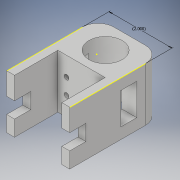
# Autodesk Inventor part: Vertical Seeder Rod spacer
Saved by Autodesk Inventor 2017 (Build 210142000, 142)
## iProperties
Created: 2017-05-29
Part Number: Vertical Seeder Rod spacer
Material: Generic
Document SubType Name: Modeling
Designer: Jon
Density: 1 g/cm^3
Appearance: Default
Author: Jon
Autodesk Inventor part; units mm, degrees
ref_plane "YZ Plane" through (0, 0, 0) normal (1, 0, 0) x (0, 1, 0)
ref_plane "XZ Plane" through (0, 0, 0) normal (0, 1, 0) x (-1, 0, 0)
ref_plane "XY Plane" through (0, 0, 0) normal (0, 0, 1) x (1, 0, 0)
sketch "Sketch1" plane through (0, 0, 0) normal (0, 0, 1) x (1, 0, 0)
  line L0 (-15.24, 10.0753) -> (16.51, 10.0753)
  line L1 (16.51, 10.0753) -> (16.51, -15.3247)
  line L2 (16.51, -15.3247) -> (-15.24, -15.3247)
  line L3 (-15.24, -15.3247) -> (-15.24, 10.0753)
  circle A0 centre (-11.43, 6.2653) radius 1.905
  circle A1 centre (-11.43, -6.4347) radius 1.905
  circle A2 centre (12.7, 6.2653) radius 1.905
  circle A3 centre (12.7, -6.4347) radius 1.905
  point P0 (0, 0)
  dimension "d0" = 31.75
  dimension "d1" = 25.4
  dimension "d10" = 3.81
  dimension "d11" = 8.89
  dimension "d12" = 3.81
  dimension "d13" = 3.81
  dimension "d14" = 8.89
  dimension "d15" = 3.81
  dimension "d16" = 3.81
  dimension "d17" = 3.81
  dimension "d18" = 3.81
  dimension "d19" = 3.81
  dimension "d20" = 3.81
  dimension "d21" = 3.81
  dimension "d22" = 8.89
  constraints: 8 end point, 4 centre point, 2 parallel, 1 horizontal, 1 perpendicular
  measures "d0" distance of L0.start L0.end
  measures "d1" distance of L0.end L1.end
  measures "d10" diameter of A0
  measures "d12" distance from line of L0 A0.centre
  measures "d13" distance from line of L3 A0.centre
  measures "d14" distance from line of L2 A1.centre
  measures "d15" diameter of A2
  measures "d16" diameter of A1
  measures "d17" diameter of A3
  measures "d18" distance from line of L3 A1.centre
  measures "d19" distance from line of L0 A2.centre
  measures "d20" distance from line of L1 A2.centre
  measures "d21" distance from line of L1 A3.centre
  measures "d22" distance from line of L2 A3.centre
extrude "Extrusion1" add sketch "Sketch1" along normal blind 6.35
sketch "Sketch2" plane through (0, 0, 6.35) normal (0, 0, 1) x (1, 0, 0)
  line L0 (-24.765, 16.4253) -> (26.035, 16.4253)
  line L1 (26.035, 16.4253) -> (26.035, -21.6747)
  line L2 (26.035, -21.6747) -> (-24.765, -21.6747)
  line L3 (-24.765, -21.6747) -> (-24.765, 16.4253)
  line L4 (16.51, -15.3247) -> (16.51, 10.0753) projected
  line L5 (-15.24, 10.0753) -> (-15.24, -15.3247) projected
  line L6 (16.51, 10.0753) -> (-15.24, 10.0753) projected
  point P0 (0, 0)
  dimension "d25" = 50.8
  dimension "d26" = 38.1
  dimension "d27" = 9.525
  dimension "d29" = 9.525
  dimension "d30" = 6.35
  constraints: 8 end point, 2 parallel, 1 horizontal, 1 perpendicular
  measures "d25" distance of L0.start L0.end
  measures "d26" distance of L0.end L1.end
  measures "d27" distance between parallel lines of L4 L1
  measures "d29" distance between parallel lines of L3 L5
  measures "d30" distance between parallel lines of L6 L0
extrude "Extrusion2" add sketch "Sketch2" along normal blind 6.35
sketch "Sketch3" plane through (0, 0, 6.35) normal (0, 0, -1) x (-1, 0, 0)
  line L0 (24.765, -21.6747) -> (24.765, 16.4253) projected
  circle A0 centre (11.43, 6.2653) radius 1.905 projected
  line L1 (24.765, 16.4253) -> (-26.035, 16.4253) projected
  circle A1 centre (11.43, -6.4347) radius 1.905 projected
  line L2 (-26.035, -21.6747) -> (24.765, -21.6747) projected
  line L3 (-26.035, 16.4253) -> (-26.035, -21.6747) projected
  point P0 (0, 0)
  point P1 (-12.7, -6.4347)
  point P2 (-12.7, 6.2653)
  dimension "d33" = 13.335
  dimension "d34" = 10.16
  dimension "d35" = 13.335
  dimension "d36" = 15.24
  dimension "d37" = 13.335
  dimension "d38" = 10.16
  dimension "d39" = 15.24
  dimension "d40" = 13.335
  constraints: 2 coincident
  measures "d33" distance from line of L0 A0.centre
  measures "d34" distance from line of L1 A0.centre
  measures "d35" distance from line of L0 A1.centre
  measures "d36" distance from line of L2 A1.centre
  measures "d37" distance from line of L3 point (-12.7, 6.265)
  measures "d38" distance from line of L1 point (-12.7, 6.265)
  measures "d39" distance from line of L2 point (-12.7, -6.435)
  measures "d40" distance from line of L3 point (-12.7, -6.435)
hole "Hole1" at (-11.43, 6.2653, 6.35) at (-11.43, -6.4347, 6.35) at (12.7, -6.4347, 6.35) at (12.7, 6.2653, 6.35) direction (0, 0, 1) diameter 3.81 end through all
sketch "Sketch4" plane through (0, 0, 12.7) normal (0, 0, 1) x (1, 0, 0)
  line L0 (26.035, 16.4253) -> (26.035, -21.6747) projected
  line L1 (26.035, 16.4253) -> (19.685, 16.4253)
  line L2 (19.685, 16.4253) -> (19.685, -21.6747)
  line L3 (19.685, -21.6747) -> (26.035, -21.6747)
  line L4 (26.035, -21.6747) -> (26.035, 16.4253)
  line L5 (-24.765, 16.4253) -> (26.035, 16.4253) projected
  line L6 (-24.765, 16.4253) -> (-18.415, 16.4253)
  line L7 (-18.415, 16.4253) -> (-18.415, -21.6747)
  line L8 (-18.415, -21.6747) -> (-24.765, -21.6747)
  line L9 (-24.765, -21.6747) -> (-24.765, 16.4253)
  point P0 (0, 0)
  dimension "d48" = 6.35
  dimension "d49" = 6.35
  constraints: 16 end point, 4 parallel, 2 horizontal, 2 perpendicular, 1 point on line
  measures "d48" distance of L2.end L3.end
  measures "d49" distance of L7.end L8.end
extrude "Extrusion3" add sketch "Sketch4" along normal blind 34.925
sketch "Sketch5" plane through (26.035, -21.6747, 6.35) normal (1, 0, 0) x (0, 0, -1)
  line L0 (-41.2903, 25.4) -> (-28.2305, 25.4)
  line L1 (-28.2305, 25.4) -> (-28.2305, 12.7)
  line L2 (-28.2305, 12.7) -> (-41.2903, 12.7)
  line L3 (-41.2903, 12.7) -> (-41.2903, 25.4)
  line L4 (0, 38.1) -> (-41.275, 38.1) projected
  point P0 (6.35, 21.6747)
  dimension "d52" = 12.7
  dimension "d53" = 12.7
  constraints: 8 end point, 2 parallel, 1 horizontal, 1 perpendicular
  measures "d52" distance between parallel lines of L4 L0
  measures "d53" distance of L2.end L0.start
extrude "Extrusion4" cut sketch "Sketch5" against normal through all
sketch "Sketch6" plane through (0, 0, 6.35) normal (0, 0, -1) x (-1, 0, 0)
  point P0 (0, 0)
sketch "Sketch7" plane through (0, 0, 6.35) normal (0, 0, -1) x (-1, 0, 0)
  line L0 (-26.035, 16.4253) -> (-26.035, -21.6747) projected
  line L1 (24.765, -21.6747) -> (18.415, -21.6747) projected
  line L2 (-26.035, 16.4253) -> (24.765, 16.4253)
  line L3 (24.765, 16.4253) -> (24.765, -21.6747)
  line L4 (24.765, -21.6747) -> (-26.035, -21.6747)
  line L5 (-26.035, -21.6747) -> (-26.035, 16.4253)
  point P0 (0, 0)
  constraints: 8 end point, 2 parallel, 1 horizontal, 1 perpendicular
extrude "Extrusion5" add sketch "Sketch7" along normal blind 32.385
sketch "Sketch8" plane through (-18.415, -21.6747, 12.7) normal (0, -1, 0) x (1, 0, 0)
  line L0 (44.45, -38.735) -> (-6.35, -38.735) projected
  line L1 (44.45, 34.925) -> (44.45, -38.735) projected
  line L2 (0, 0) -> (38.1, 0) projected
  line L3 (-6.35, 34.925) -> (-6.35, -38.735) projected
  point P0 (18.415, -12.7)
  point P1 (19.05, -19.3675)
  dimension "d60" = 19.3675
  dimension "d61" = 25.4
  dimension "d62" = 19.3675
  dimension "d63" = 25.4
  measures "d60" distance from line of L0 point (19.05, -19.367)
  measures "d61" distance from line of L1 point (19.05, -19.367)
  measures "d62" distance from line of L2 point (19.05, -19.367)
  measures "d63" distance from line of L3 point (19.05, -19.367)
hole "Hole2" at (0.635, -21.6747, -6.6675) direction (0, 1, 0) diameter 26.797 end through all
fillet "Fillet3" radius 12.7 2 edges at (-24.765, -2.6247, -26.035) (26.035, -2.6247, -26.035)
sketch "Sketch9" plane through (0, 0, 12.7) normal (0, 0, 1) x (1, 0, 0)
  circle A0 centre (12.7, -6.4347) radius 1.905
  circle A1 centre (-11.43, -6.4347) radius 1.905
  circle A2 centre (-11.43, 6.2653) radius 1.905
  line L0 (-18.415, -21.6747) -> (19.685, -21.6747) projected
  line L1 (26.035, 3.7253) -> (26.035, -8.9747) projected
  circle A3 centre (12.7, 6.2653) radius 1.905 projected
  circle A4 centre (-11.43, -6.4347) radius 1.905 projected
  circle A5 centre (12.7, 6.2653) radius 1.905
  line L2 (19.685, 16.4253) -> (-18.415, 16.4253) projected
  point P0 (0, 0)
  dimension "d73" = 15.24
  dimension "d74" = 13.335
  dimension "d75" = 12.7
  dimension "d76" = 24.13
  dimension "d77" = 24.13
  dimension "d78" = 3.81
  dimension "d79" = 3.81
  dimension "d80" = 12.7
  dimension "d81" = 3.81
  dimension "d82" = 10.16
  dimension "d83" = 24.13
  constraints: 4 centre point, 1 coincident, 1 concentric
  measures "d73" distance from line of L0 A0.centre
  measures "d74" distance from line of L1 A0.centre
  measures "d75" distance of A3.centre A0.centre
  measures "d76" distance of A4.centre A0.centre
  measures "d77" distance of A0.centre A1.centre
  measures "d78" diameter of A0
  measures "d79" diameter of A1
  measures "d80" distance of A1.centre A2.centre
  measures "d81" diameter of A2
  measures "d82" distance from line of L2 A2.centre
  measures "d83" distance of A3.centre A2.centre
extrude "Extrusion6" cut sketch "Sketch9" against normal blind 19.05
sketch "Sketch10" plane through (26.035, 3.7253, 47.625) normal (1, 0, 0) x (0, 0, -1)
  line L0 (41.275, 8.89) -> (53.975, 8.89)
  line L1 (53.975, 8.89) -> (53.975, -16.51)
  line L2 (53.975, -16.51) -> (41.275, -16.51)
  line L3 (41.275, -16.51) -> (41.275, 8.89)
  line L4 (34.925, -25.4) -> (34.925, 12.7) projected
  line L5 (0, 12.7) -> (60.96, 12.7) projected
  point P0 (47.625, -3.7253)
  dimension "d86" = 12.7
  dimension "d87" = 25.4
  dimension "d88" = 6.35
  dimension "d91" = 3.81
  constraints: 8 end point, 2 parallel, 1 horizontal, 1 perpendicular
  measures "d86" distance of L0.start L0.end
  measures "d87" distance of L0.end L1.end
  measures "d88" distance between parallel lines of L3 L4
  measures "d91" distance between parallel lines of L5 L0
extrude "Extrusion7" cut sketch "Sketch10" against normal through all
thicken "Thicken1" operation add thickness 5.08 both sides no extend neighbours yes toward (0, 1, 0) faces at (-22.6483, 16.4253, 15.6633)
sketch "Sketch11" plane through (-18.415, 21.5053, 12.7) normal (0, 1, 0) x (1, 0, 0)
  point P0 (18.415, 12.7)
sketch "Sketch12" plane through (-24.765, -21.6747, 47.625) normal (-1, 0, 0) x (0, 0, 1)
  line L0 (-60.96, 43.18) -> (0, 43.18) projected
  line L1 (0, 0) -> (-60.96, 0) projected
  point P0 (-47.625, 21.6747)
sketch "Sketch13" plane through (-18.415, 21.5053, 12.7) normal (0, 1, 0) x (1, 0, 0)
  line L0 (44.45, -34.925) -> (44.45, 26.035) projected
  line L1 (-6.35, 26.035) -> (-6.35, -34.925) projected
  point P0 (18.415, 12.7)
  dimension "d95" = 50.8
  measures "d95" distance between parallel lines of L0 L1
equation "\"d12\" = d13"
equation "\"d15\" = d10"
equation "\"d16\" = d10"
equation "\"d17\" = d10"
equation "\"d19\" = d13"
equation "\"d20\" = d13"
equation "\"d21\" = d20"
equation "\"d22\" = d14"
equation "\"d37\" = d33"
equation "\"d38\" = d34"
equation "\"d39\" = d36"
equation "\"d40\" = d35"
equation "\"d77\" = d76"
equation "\"d79\" = d78"
body "Solid1"
